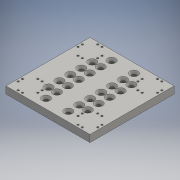
# Autodesk Inventor part: 6dof_plate
Saved by Autodesk Inventor 2016 (Build 200138000, 138)
## iProperties
Created: 2016-07-08
Part Number: 6dof_plate
Material: Generic
Document SubType Name: Modeling
Designer: kam42
Density: 1 g/cm^3
Appearance: Default
Author: kam42
Autodesk Inventor part; units mm, degrees
ref_plane "YZ Plane" through (0, 0, 0) normal (1, 0, 0) x (0, 1, 0)
ref_plane "XZ Plane" through (0, 0, 0) normal (0, 1, 0) x (-1, 0, 0)
ref_plane "XY Plane" through (0, 0, 0) normal (0, 0, 1) x (1, 0, 0)
sketch "Sketch1" plane through (0, 0, 0) normal (0, 0, 1) x (1, 0, 0)
  line L0 (-37.5, -37.5) -> (37.5, -37.5)
  line L1 (37.5, -37.5) -> (37.5, 37.5)
  line L2 (37.5, 37.5) -> (-37.5, 37.5)
  line L3 (-37.5, 37.5) -> (-37.5, -37.5)
  line L4 (-37.5, -37.5) -> (37.5, 37.5) construction
  line L5 (37.5, -37.5) -> (-37.5, 37.5) construction
  point P0 (0, 0)
  dimension "d0" = 75
  dimension "d1" = 75
  constraints: 12 end point, 2 midpoint, 2 parallel, 1 horizontal, 1 perpendicular
  measures "d0" distance of L1.end L2.end
  measures "d1" distance of L0.end L1.end
extrude "Extrusion1" add sketch "Sketch1" along normal blind 6.35
sketch "Sketch2" plane through (0, 0, 6.35) normal (0, 0, 1) x (1, 0, 0)
  line L0 (-15.91, 15.91) -> (-37.5, 15.91) construction
  line L1 (-37.5, 15.91) -> (-37.5, 37.5) construction
  line L2 (-37.5, 37.5) -> (-15.91, 37.5) construction
  line L3 (-15.91, 37.5) -> (-15.91, 15.91) construction
  line L4 (-15.91, 15.91) -> (-37.5, 37.5) construction
  line L5 (-37.5, 15.91) -> (-15.91, 37.5) construction
  line L6 (-15.91, -15.91) -> (-15.91, -37.5) construction
  line L7 (-15.91, -37.5) -> (-37.5, -37.5) construction
  line L8 (-37.5, -37.5) -> (-37.5, -15.91) construction
  line L9 (-37.5, -15.91) -> (-15.91, -15.91) construction
  line L10 (-15.91, -15.91) -> (-37.5, -37.5) construction
  line L11 (-15.91, -37.5) -> (-37.5, -15.91) construction
  line L12 (15.91, -15.91) -> (37.5, -15.91) construction
  line L13 (37.5, -15.91) -> (37.5, -37.5) construction
  line L14 (37.5, -37.5) -> (15.91, -37.5) construction
  line L15 (15.91, -37.5) -> (15.91, -15.91) construction
  line L16 (15.91, -15.91) -> (37.5, -37.5) construction
  line L17 (37.5, -15.91) -> (15.91, -37.5) construction
  line L18 (15.91, 15.91) -> (15.91, 37.5) construction
  line L19 (15.91, 37.5) -> (37.5, 37.5) construction
  line L20 (37.5, 37.5) -> (37.5, 15.91) construction
  line L21 (37.5, 15.91) -> (15.91, 15.91) construction
  line L22 (15.91, 15.91) -> (37.5, 37.5) construction
  line L23 (15.91, 37.5) -> (37.5, 15.91) construction
  line L24 (37.5, 37.5) -> (-37.5, 37.5) projected
  line L25 (-37.5, 37.5) -> (-37.5, -37.5) projected
  point P0 (0, 0)
  point P1 (-26.705, 26.705)
  point P2 (-24.8, 35.468)
  point P3 (-35.468, 24.8)
  point P4 (-35.468, 28.61)
  point P5 (-24.8, 17.942)
  point P6 (-28.61, 17.942)
  point P7 (-17.942, 28.61)
  point P8 (-17.942, 24.8)
  point P9 (-28.61, 35.468)
  point P10 (-26.705, -26.705)
  point P11 (-35.468, -28.61)
  point P12 (-24.8, -17.942)
  point P13 (-28.61, -17.942)
  point P14 (-17.942, -28.61)
  point P15 (-17.942, -24.8)
  point P16 (-28.61, -35.468)
  point P17 (-24.8, -35.468)
  point P18 (-35.468, -24.8)
  point P19 (26.705, -26.705)
  point P20 (28.61, -35.468)
  point P21 (17.942, -24.8)
  point P22 (17.942, -28.61)
  point P23 (28.61, -17.942)
  point P24 (24.8, -17.942)
  point P25 (35.468, -28.61)
  point P26 (35.468, -24.8)
  point P27 (24.8, -35.468)
  point P28 (26.705, 26.705)
  point P29 (35.468, 28.61)
  point P30 (24.8, 17.942)
  point P31 (28.61, 17.942)
  point P32 (17.942, 28.61)
  point P33 (17.942, 24.8)
  point P34 (28.61, 35.468)
  point P35 (24.8, 35.468)
  point P36 (35.468, 24.8)
  dimension "d4" = 21.59
  dimension "d5" = 21.59
  dimension "d6" = 2.032
  dimension "d7" = 12.7
  dimension "d10" = 360
  dimension "d15" = 360
  constraints: 48 end point, 8 midpoint, 2 collinear, 2 parallel, 1 horizontal, 1 perpendicular, 1 symmetric about line, 86 other
  measures "d4" distance of L1.end L2.end
  measures "d5" distance of L0.end L1.end
  measures "d6" distance from line of L2 point (-24.8, 35.468)
  measures "d7" distance from line of point (-24.8, 35.468) L1
hole "Hole1" at (-24.8, 35.468, 6.35) at (-35.468, 24.8, 6.35) at (-35.468, 28.61, 6.35) at (-24.8, 17.942, 6.35) at (-28.61, 17.942, 6.35) at (-17.942, 28.61, 6.35) at (-17.942, 24.8, 6.35) at (-28.61, 35.468, 6.35) at (-35.468, -28.61, 6.35) at (-24.8, -17.942, 6.35) at (-28.61, -17.942, 6.35) at (-17.942, -28.61, 6.35) at (-17.942, -24.8, 6.35) at (-28.61, -35.468, 6.35) at (-24.8, -35.468, 6.35) at (-35.468, -24.8, 6.35) at (28.61, -35.468, 6.35) at (17.942, -24.8, 6.35) at (17.942, -28.61, 6.35) at (28.61, -17.942, 6.35) at (24.8, -17.942, 6.35) at (35.468, -28.61, 6.35) at (35.468, -24.8, 6.35) at (24.8, -35.468, 6.35) at (35.468, 28.61, 6.35) at (24.8, 17.942, 6.35) at (28.61, 17.942, 6.35) at (17.942, 28.61, 6.35) at (17.942, 24.8, 6.35) at (28.61, 35.468, 6.35) at (24.8, 35.468, 6.35) at (35.468, 24.8, 6.35) direction (0, 0, -1) diameter 1.694 depth 6.637 tip angle 118 thread size "2-56 UNC" class "2B" standard "ANSI Unified Screw Threads"
sketch "Sketch3" plane through (0, 0, 6.35) normal (0, 0, 1) x (1, 0, 0)
  line L0 (-37.5, 37.5) -> (-37.5, -37.5) construction
  line L1 (37.5, -37.5) -> (37.5, 37.5) construction
  line L2 (37.5, 37.5) -> (-37.5, 37.5) construction
  line L3 (-37.5, 37.5) -> (-37.5, -37.5) construction
  line L4 (-17.5, -19.5) -> (17.5, -19.5) construction
  line L5 (37.5, 37.5) -> (-37.5, 37.5) construction
  line L6 (-37.5, -37.5) -> (37.5, -37.5) construction
  circle A0 centre (-17.942, 24.8) radius 0.847 projected
  circle A1 centre (-17.942, -24.8) radius 0.847 projected
  point P0 (-17.5, -9.75)
  point P1 (17.5, -9.75)
  point P2 (-17.5, 0)
  point P3 (17.5, 0)
  point P4 (-17.5, 9.75)
  point P5 (17.5, 9.75)
  point P6 (-17.5, 19.5)
  point P7 (17.5, 19.5)
  dimension "d67" = 35
  dimension "d97" = 18
  dimension "d114" = 9.75
  constraints: 2 end point, 1 horizontal, 1 vertical, 8 other
  measures "d67" distance of L4.end L4.start
  measures "d97" distance between parallel lines of L6 L4
  measures "d114" distance of L4.start point (-17.5, -9.75)
hole "Hole7" at (-17.5, -19.5, 6.35) at (17.5, -19.5, 6.35) at (-17.5, -9.75, 6.35) at (17.5, -9.75, 6.35) at (-17.5, 0, 6.35) at (17.5, 0, 6.35) at (-17.5, 9.75, 6.35) at (17.5, 9.75, 6.35) at (-17.5, 19.5, 6.35) at (17.5, 19.5, 6.35) direction (0, 0, -1) diameter 3.797 depth 10.979 tip angle 118 countersink diameter 7.087 countersink angle 82 clearance for "Flat Head Machine Screw (82)" size "#6" standard "Ansi Unified Screw Threads"
sketch "Sketch4" plane through (0, 0, 6.35) normal (0, 0, 1) x (1, 0, 0)
  circle A0 centre (-17.5, -19.5) radius 1.8985 construction
  circle A1 centre (17.5, -19.5) radius 1.8985 construction
  circle A2 centre (17.5, -19.5) radius 1.8985 construction
  line L0 (-17.5, -19.5) -> (17.5, -19.5) construction
  line L1 (0, 0) -> (0, -37.5) construction
  line L2 (-37.5, -37.5) -> (37.5, -37.5) construction
  point P0 (-10, -19.5)
  point P1 (10, -19.5)
  point P2 (-10, -9.75)
  point P3 (10, -9.75)
  point P4 (-10, 0)
  point P5 (10, 0)
  point P6 (-10, 9.75)
  point P7 (10, 9.75)
  point P8 (-10, 19.5)
  point P9 (10, 19.5)
  point P10 (-10, 29.25)
  point P11 (10, 29.25)
  point P12 (-10, -29.25)
  point P13 (10, -29.25)
  point P14 (-10, -19.5)
  point P15 (10, -19.5)
  point P16 (-10, -9.75)
  point P17 (10, -9.75)
  point P18 (-10, 0)
  point P19 (10, 0)
  point P20 (-10, 9.75)
  point P21 (10, 9.75)
  point P22 (-10, 19.5)
  point P23 (10, 19.5)
  dimension "d126" = 10
  dimension "d129" = 9.75
  dimension "d132" = 9.75
  constraints: 4 end point, 2 vertical, 1 horizontal, 1 midpoint, 1 point on line, 1 symmetric about line, 22 other
  measures "d126" distance from line of point (-10, -19.5) L1
  measures "d129" distance of point (-10, -19.5) point (-10, -9.75)
  measures "d132" distance of point (-10, -19.5) point (-10, -29.25)
hole "Hole8" at (-10, -19.5, 6.35) at (10, -19.5, 6.35) at (-10, -9.75, 6.35) at (10, -9.75, 6.35) at (-10, 0, 6.35) at (10, 0, 6.35) at (-10, 9.75, 6.35) at (10, 9.75, 6.35) at (-10, 19.5, 6.35) at (10, 19.5, 6.35) at (-10, 29.25, 6.35) at (10, 29.25, 6.35) at (-10, -29.25, 6.35) at (10, -29.25, 6.35) direction (0, 0, -1) diameter 3.797 depth 10.979 tip angle 118 countersink diameter 7.087 countersink angle 82 clearance for "Flat Head Machine Screw (82)" size "#6" standard "Ansi Unified Screw Threads"
body "Solid1"
